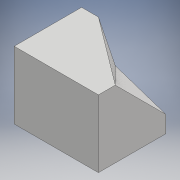
# Autodesk Inventor part: 24
Saved by Autodesk Inventor 2017 (Build 210142000, 142)
## iProperties
Part Number: 24
Material: 一般
Document SubType Name: Modeling
Designer: Brian
Density: 1 g/cm^3
Appearance: 預設
Author: Brian
Autodesk Inventor part; units mm, degrees
ref_plane "YZ Plane" through (0, 0, 0) normal (1, 0, 0) x (0, 1, 0)
sketch "草圖1" plane through (0, 0, 0) normal (0, 1, 0) x (-1, 0, 0)
  line L0 (0, 0) -> (-50, 0)
  line L1 (-50, 0) -> (-50, -40)
  line L2 (-50, -40) -> (0, -40)
  line L3 (0, -40) -> (0, 0)
  dimension "d0" = 40
  dimension "d1" = 50
  constraints: 8 end point, 2 parallel, 1 horizontal, 1 perpendicular
  measures "d0" distance of L2.end L0.start
  measures "d1" distance of L1.end L2.end
extrude "擠出1" add sketch "草圖1" along normal blind 40
sketch "草圖2" plane through (0, 0, 0) normal (0, 0, 1) x (1, 0, 0)
  line L0 (50, 10) -> (10, 40)
  line L1 (0, 40) -> (50, 40) projected
  line L2 (50, 0) -> (50, 40) projected
  point P0 (0, 0)
  dimension "d4" = 30
  dimension "d5" = 40
  constraints: 2 end point, 2 point on line
  measures "d4" vertical distance of L0.start L0.end
  measures "d5" horizontal distance of L0.start L0.end
sketch "草圖3" plane through (0, 40, 0) normal (0, 1, 0) x (1, 0, 0)
  line L0 (0, 0) -> (50, 0) projected
  line L1 (50, 0) -> (50, 40) projected
  point P0 (20, 20)
  dimension "d6" = 20
  dimension "d7" = 30
  measures "d6" distance from line of L0 point (20, 20)
  measures "d7" distance from line of L1 point (20, 20)
ref_plane "工作平面1" through (20, 40, -20) normal (0.5747, 0.7663, 0.2873) x (-0.4472, 0, 0.8944)
sketch "草圖4" plane through (20, 40, -20) normal (0.5747, 0.7663, 0.2873) x (-0.4472, 0, 0.8944)
  line L0 (0, 0) -> (4.4721, 46.6905)
  line L1 (4.4721, 46.6905) -> (47.828, 42.5377)
  line L2 (47.828, 42.5377) -> (43.3559, -4.1527)
  line L3 (43.3559, -4.1527) -> (0, 0)
  point P0 (26.8328, 18.8475)
  constraints: 8 end point, 2 parallel, 1 perpendicular
extrude "擠出2" cut sketch "草圖4" along normal blind 40
sketch "草圖5" plane through (50, 0, 0) normal (1, 0, 0) x (0, 0, -1)
  line L0 (2.1429, 40) -> (0, 10) projected
  line L1 (0, 10) -> (30, 40)
  line L2 (40, 40) -> (0, 40) projected
  point P0 (0, 0)
  dimension "d10" = 30
  constraints: 2 end point, 1 point on line
  measures "d10" horizontal distance of L0.end L1.end
ref_plane "工作平面2" through (50, 40, -30) normal (-0.2294, -0.6882, -0.6882) x (0, -0.7071, 0.7071)
sketch "草圖6" plane through (50, 40, -30) normal (-0.2294, -0.6882, -0.6882) x (0, -0.7071, 0.7071)
  line L0 (7.0711, 30.8221) -> (19.698, 4.519) projected
  line L1 (19.698, 4.519) -> (42.4264, 0) projected
  line L2 (7.0711, 30.8221) -> (42.4264, 0)
  line L3 (42.4264, 0) -> (18.1406, -27.8578)
  line L4 (18.1406, -27.8578) -> (-17.2148, 2.9643)
  line L5 (-17.2148, 2.9643) -> (7.0711, 30.8221)
  point P0 (49.4975, 47.0442)
  constraints: 8 end point, 2 parallel, 1 perpendicular
extrude "擠出3" cut sketch "草圖6" against normal blind 40
